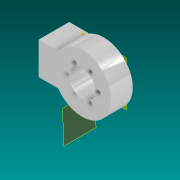
# Autodesk Inventor part: as4mount
Saved by Autodesk Inventor 2020.3 (Build 243373000, 373)
## iProperties
Created: 2020-05-24
Part Number: as4mount
Material: Aluminum 6061
Document SubType Name: Modeling
Designer: Svend
Density: 2.7 g/cm^3
Appearance: Aluminum - Polished
Author: Svend
Autodesk Inventor part; units mm, degrees
ref_plane "YZ Plane" through (0, 0, 0) normal (1, 0, 0) x (0, 1, 0)
ref_plane "XZ Plane" through (0, 0, 0) normal (0, 1, 0) x (-1, 0, 0)
ref_plane "XY Plane" through (0, 0, 0) normal (0, 0, 1) x (1, 0, 0)
ref_plane "Work Plane1" through (0, 0, 0) normal (0, 0, 1) x (1, 0, 0)
sketch "Sketch1" plane through (0, 0, 0) normal (0, 0, 1) x (1, 0, 0)
  circle A0 centre (-9.7177, -19.0526) radius 1.5 projected
  circle A1 centre (-9.7177, 19.0526) radius 1.5 projected
  circle A2 centre (-42.7177, 0) radius 1.5 projected
  circle A3 centre (-31.7177, 19.0526) radius 1.5 projected
  circle A4 centre (1.2823, 0) radius 1.5 projected
  circle A5 centre (-31.7177, -19.0526) radius 1.5 projected
  circle A6 centre (-20.7177, 0) radius 18.5 projected
  circle A7 centre (-20.7177, 0) radius 28.489 projected
  arc A8 (-0.9731, 34.7871) -> (0.731, -33.7631) centre (-20.7177, 0) ccw projected
  circle A9 centre (-20.7177, 0) radius 40 projected
  point P0 (0, 0)
extrude "Extrusion1" add sketch "Sketch1" along normal blind 30 contours A7 | A9 A8
sketch "Sketch2" plane through (-20.7177, 0, 30) normal (0, 0, 1) x (1, 0, 0)
  circle A0 centre (0, 0) radius 40 projected
  circle A1 centre (0, 0) radius 40 projected
  line L0 (-33.0719, -22.5) -> (-60, -22.5)
  line L1 (-60, -22.5) -> (-60, 22.5)
  line L2 (-60, 22.5) -> (-33.0719, 22.5)
  circle A2 centre (-22, 0) radius 1.5 projected
  line L3 (0, 0) -> (-22, 0)
  point P0 (20.7177, 0)
  point P1 (-60, 0)
  dimension "d2" = 60
  dimension "d3" = 45
  constraints: 8 end point, 2 horizontal, 2 perpendicular, 2 point on circle, 1 horizontal alignment, 1 midpoint, 1 parallel
  measures "d2" distance from line of A0.centre L1
  measures "d3" distance between parallel lines of L0 L2
ref_plane "Work Plane2" through (-100.6874, -79.9697, -0.1) normal (0, 0, 1) x (0.9996912, 0.0248509, 0)
extrude "Extrusion2" add sketch "Sketch2" against normal up to surface (30.1 mm away) contours A0 L0 L1 L2
sketch "Sketch3" plane through (-53.7896, -22.5, -0.1) normal (0, 0, -1) x (-1, 0, 0)
  arc A0 (0, 0) -> (0, 45) centre (-33.0719, 22.5) ccw projected
  line L0 (0, 0) -> (26.9281, 0) projected
  line L1 (26.9281, 0) -> (26.9281, 45) projected
  line L2 (26.9281, 45) -> (0, 45) projected
  point P0 (-53.7896, 22.5)
extrude "Extrusion3" add sketch "Sketch3" along normal blind 12
sketch "Sketch4" plane through (-80.7177, -22.5, 30) normal (-1, 0, 0) x (0, 0, 1)
  ellipse E0 centre (-20.8497, 21.2127) end of major axis (-33.3497, 21.2127) minor radius 12.4961 projected
  point P0 (-30, 22.5)
  constraints: 1 other
extrude "Extrusion4" cut sketch "Sketch4" against normal blind 7
sketch "Sketch5" plane through (-73.7177, -22.5, 30) normal (-1, 0, 0) x (0, 0, 1)
  ellipse E0 centre (-20.8497, 21.2177) end of major axis (-33.5497, 21.2177) minor radius 12.6961 projected
  circle A0 centre (-20.8497, 21.2177) radius 11
  point P0 (-30, 22.5)
  dimension "d10" = 22
  constraints: 1 centre point, 1 coincident, 1 other
  measures "d10" diameter of A0
extrude "Extrusion5" cut sketch "Sketch5" against normal blind 7 contours A0
chamfer "Chamfer1" distance 2 angle 45 6 edges at (-33.2177, 19.0526, 30) (-11.2177, 19.0526, 30) (-0.2177, 0, 30) (-11.2177, -19.0526, 30) (-33.2177, -19.0526, 30) (-44.2177, 0, 30)
ref_plane "Work Plane3" through (-45.4739, -64.3267, 9.15) normal (-0.9996912, -0.0248509, 0) x (0, 0, -1)
body "Solid1"
